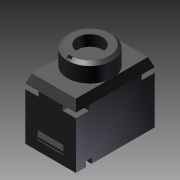
# Autodesk Inventor part: GP-body
Saved by Autodesk Inventor 2011 SP1 (Build 150282100, 282)
## iProperties
Created: 2013-12-24
Part Number: GP-body
Catalog Web Link: www.cadenas.de
Description: G Series - Process Sealed Ultra-Miniature Toggles -body-
Vendor: NKKSWITCHES
Document SubType Name: Modeling
Designer: PARTuser1
Manufacturer: NKKSWITCHES
Density: 1 g/cm^3
Category: PARTsolutions
Company: NKKSWITCHES
Title: GP-body
Author: Cadenas PARTsolutions
PSOL_IDENT_0: {$CADENAS_DATA\23d-libs\nkkswitches\toggle\g\parts\g_body.prj},211 {VTYP=3D},{NB=GP-body},{LINA=GP-b
PSOL_IDENT_1: ody},{NN=G Series - Process Sealed Ultra-Miniature Toggles -body},{DATE=12.03.2009 08:21:56},{GEOMDA
PSOL_IDENT_2: TE=12.03.2009 07:17:00},{VERSION=},{LINEID=10},{LINESUBID=-1},{WBVAR=TRMNLS}  {NB=GP-body},{LINA=GP-
PSOL_IDENT_3: body},{KT=DUMMY},{PN=GP},{SRS=G},{TRMNLS=P}
CNS_NN: G Series - Process Sealed Ultra-Miniature Toggles -body
CNS_NB: GP-body
CNS_NBSYN: $PN.-body
CNS_LINA: GP-body
CNS_PN: GP
CNS_SRS: G
CNS_TRMNLS: P - Straight
SUPPLIER: NKKSWITCHES
ARTICLENO: GP-body
BOMINFO: GP-body
CREATOR: CADENAS GmbH
Autodesk Inventor part; units mm, degrees
sketch "Sketch_1" plane through (0, 0, 0) normal (0, 1, 0) x (-1, 0, 0)
  line L0 (2.2479, 3.5052) -> (-2.2479, 3.5052)
  line L1 (-2.2479, 3.5052) -> (-2.2479, -3.5052)
  line L2 (-2.2479, -3.5052) -> (2.2479, -3.5052)
  line L3 (2.2479, -3.5052) -> (2.2479, 3.5052)
  constraints: 8 end point
extrude "Extrusion1" add sketch "Sketch_1" against normal blind 5.4102
sketch "Sketch_2" plane through (0, 0, 0) normal (0, 0, 1) x (1, 0, 0)
  line L0 (-2.2479, -0.7874) -> (-1.9456, 0)
  line L1 (-1.9456, 0) -> (1.9456, 0)
  line L2 (1.9456, 0) -> (2.2479, -0.7874)
  line L3 (2.2479, -0.7874) -> (2.2479, 0.127)
  line L4 (2.2479, 0.127) -> (-2.2479, 0.127)
  line L5 (-2.2479, 0.127) -> (-2.2479, -0.7874)
  constraints: 12 end point
extrude "Extrusion2" cut sketch "Sketch_2" along normal mid plane 7.0104
sketch "Sketch_3" plane through (0, 0, 0) normal (1, 0, 0) x (0, 1, 0)
  line L0 (-0.7874, 3.5052) -> (0, 3.2029)
  line L1 (0, 3.2029) -> (0, -3.2029)
  line L2 (0, -3.2029) -> (-0.7874, -3.5052)
  line L3 (-0.7874, -3.5052) -> (0.127, -3.5052)
  line L4 (0.127, -3.5052) -> (0.127, 3.5052)
  line L5 (0.127, 3.5052) -> (-0.7874, 3.5052)
  constraints: 12 end point
extrude "Extrusion3" cut sketch "Sketch_3" along normal mid plane 4.4958
sketch "Sketch_4" plane through (0, -0.9906, 0) normal (0, 1, 0) x (1, 0, 0)
  line L0 (-2.5256, 3.7556) -> (-2.5256, -3.7297)
  line L1 (-2.5256, -3.7297) -> (2.532, -3.7297)
  line L2 (2.532, -3.7297) -> (2.532, 3.7556)
  line L3 (2.532, 3.7556) -> (-2.5256, 3.7556)
  line L4 (-2.2479, 2.3368) -> (-2.2479, -2.3368)
  line L5 (-2.2479, -2.3368) -> (-1.0668, -2.3368)
  line L6 (-1.0668, -2.3368) -> (-1.0668, -3.5052)
  line L7 (-1.0668, -3.5052) -> (1.0668, -3.5052)
  line L8 (1.0668, -3.5052) -> (1.0668, -2.3368)
  line L9 (1.0668, -2.3368) -> (2.2479, -2.3368)
  line L10 (2.2479, -2.3368) -> (2.2479, 2.3368)
  line L11 (2.2479, 2.3368) -> (1.0668, 2.3368)
  line L12 (1.0668, 2.3368) -> (1.0668, 3.5052)
  line L13 (1.0668, 3.5052) -> (-1.0668, 3.5052)
  line L14 (-1.0668, 3.5052) -> (-1.0668, 2.3368)
  line L15 (-1.0668, 2.3368) -> (-2.2479, 2.3368)
  constraints: 32 end point
extrude "Extrusion4" cut sketch "Sketch_4" along normal mid plane 0.4318
sketch "Sketch_5" plane through (0, 0, 0) normal (1, 0, 0) x (0, 1, 0)
  line L0 (0, 0) -> (1.6002, 0)
  line L1 (0.635, 0) -> (0.635, -1.1176)
  line L2 (0.635, -1.1176) -> (1.6002, -1.1176)
  line L3 (1.6002, -1.1176) -> (1.6002, -1.7399)
  line L4 (1.6002, -1.7399) -> (1.3462, -1.9939)
  line L5 (1.3462, -1.9939) -> (0, -1.9939)
  line L6 (0, -1.9939) -> (0, 0)
  line L7 (0, 0) -> (0.635, 0)
  constraints: 16 end point
revolve "Revolution1" add sketch "Sketch_5" angle 360 about axis through (0, 0, 0) along (0, -1, 0)
sketch "Sketch_6" plane through (0, -5.4102, 0) normal (0, 1, 0) x (1, 0, 0)
  line L0 (-2.6354, 3.6285) -> (-2.6354, -3.6285)
  line L1 (-2.6354, -3.6285) -> (2.6743, -3.6285)
  line L2 (2.6743, -3.6285) -> (2.6743, 3.6285)
  line L3 (2.6743, 3.6285) -> (-2.6354, 3.6285)
  line L4 (-2.2479, -3.5052) -> (2.2479, -3.5052)
  line L5 (2.2479, -3.5052) -> (2.2479, -2.6162)
  line L6 (2.2479, -2.6162) -> (1.7399, -2.6162)
  line L7 (1.7399, -2.6162) -> (1.7399, -2.1082)
  line L8 (1.7399, -2.1082) -> (2.2479, -2.1082)
  line L9 (2.2479, -2.1082) -> (2.2479, 3.5052)
  line L10 (2.2479, 3.5052) -> (-2.2479, 3.5052)
  line L11 (-2.2479, 3.5052) -> (-2.2479, -2.1082)
  line L12 (-2.2479, -2.1082) -> (-1.7399, -2.1082)
  line L13 (-1.7399, -2.1082) -> (-1.7399, -2.6162)
  line L14 (-1.7399, -2.6162) -> (-2.2479, -2.6162)
  line L15 (-2.2479, -2.6162) -> (-2.2479, -3.5052)
  constraints: 32 end point
extrude "Extrusion5" cut sketch "Sketch_6" along normal blind 0.4572
sketch "Sketch_7" plane through (0, -5.4102, 0) normal (0, 1, 0) x (1, 0, 0)
  line L0 (-1.8669, 2.8702) -> (-1.8669, -2.8702)
  arc A0 (-1.8669, -2.8702) -> (-1.6129, -3.1242) centre (-1.6129, -2.8702) ccw
  line L1 (-1.6129, -3.1242) -> (1.6129, -3.1242)
  arc A1 (1.6129, -3.1242) -> (1.8669, -2.8702) centre (1.6129, -2.8702) ccw
  line L2 (1.8669, -2.8702) -> (1.8669, 2.8702)
  arc A2 (1.8669, 2.8702) -> (1.6129, 3.1242) centre (1.6129, 2.8702) ccw
  line L3 (1.6129, 3.1242) -> (-1.6129, 3.1242)
  arc A3 (-1.6129, 3.1242) -> (-1.8669, 2.8702) centre (-1.6129, 2.8702) ccw
  constraints: 8 end point, 8 point on circle, 4 centre point
extrude "Extrusion6" cut sketch "Sketch_7" along normal blind 0.0508
sketch "Sketch_11" plane through (0, 1.6002, 0) normal (0, 1, 0) x (1, 0, 0)
  line L0 (-0.1905, -1.7145) -> (-0.1905, -2.0955)
  line L1 (-0.1905, -2.0955) -> (0.1905, -2.0955)
  line L2 (0.1905, -2.0955) -> (0.1905, -1.7145)
  line L3 (0.1905, -1.7145) -> (-0.1905, -1.7145)
  constraints: 8 end point
extrude "Extrusion7" cut sketch "Sketch_11" against normal blind 0.254
sketch "Sketch_13" plane through (0, 0, 0) normal (0, 0, 1) x (1, 0, 0)
  line L0 (-1.143, -3.81) -> (-1.143, -4.572)
  line L1 (-1.143, -4.572) -> (1.143, -4.572)
  line L2 (1.143, -4.572) -> (1.143, -3.81)
  line L3 (1.143, -3.81) -> (-1.143, -3.81)
  constraints: 8 end point
extrude "Extrusion8" cut sketch "Sketch_13" along normal mid plane 15.24
sketch "Sketch_14" plane through (0, 0, 0) normal (1, 0, 0) x (0, 1, 0)
  line L0 (-4.3688, 3.4544) -> (-4.572, 3.4544)
  line L1 (-4.572, 3.4544) -> (-4.572, -3.4544)
  line L2 (-4.572, -3.4544) -> (-4.3688, -3.4544)
  line L3 (-4.3688, -3.4544) -> (-3.81, -3.1318)
  line L4 (-3.81, -3.1318) -> (-3.81, 3.1318)
  line L5 (-3.81, 3.1318) -> (-4.3688, 3.4544)
  constraints: 12 end point
extrude "Extrusion9" add sketch "Sketch_14" along normal mid plane 2.286
ref_plane "to_actuator_XY" through (0, 0, 0) normal (0, -1, 0) x (1, 0, 0)
ref_plane "to_actuator_YZ" through (0, 0, 0) normal (1, 0, 0) x (0, 0, 1)
ref_plane "to_actuator_ZX" through (0, 0, 0) normal (0, 0, 1) x (0, -1, 0)
ref_plane "to_dummy_XY" through (0, 0, 0) normal (0, -1, 0) x (1, 0, 0)
ref_plane "to_dummy_YZ" through (0, 0, 0) normal (1, 0, 0) x (0, 0, 1)
ref_plane "to_dummy_ZX" through (0, 0, 0) normal (0, 0, 1) x (0, -1, 0)
ref_plane "to_trmnl_hold_XY" through (0, -0.9906, 0) normal (0, 1, 0) x (1, 0, 0)
ref_plane "to_trmnl_hold_YZ" through (0, -0.9906, 0) normal (1, 0, 0) x (0, 0, -1)
ref_plane "to_trmnl_hold_ZX" through (0, -0.9906, 0) normal (0, 0, -1) x (0, 1, 0)
ref_plane "to_trmnls_XY" through (0, -4.9022, 0) normal (0, 1, 0) x (1, 0, 0)
ref_plane "to_trmnls_YZ" through (0, -4.9022, 0) normal (1, 0, 0) x (0, 0, -1)
ref_plane "to_trmnls_ZX" through (0, -4.9022, 0) normal (0, 0, -1) x (0, 1, 0)
body "Solid1"
